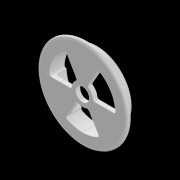
# Autodesk Inventor part: ToroidalCap
Saved by Autodesk Inventor 2020.4 (Build 244396010, 396A)
## iProperties
Created: 2022-09-18
Part Number: ToroidalCap
Material: Generic
Document SubType Name: Modeling
Designer: Val
Density: 1 g/cm^3
Appearance: Default
Author: Val
Autodesk Inventor part; units mm, degrees
ref_plane "YZ Plane" through (0, 0, 0) normal (1, 0, 0) x (0, 1, 0)
ref_plane "XZ Plane" through (0, 0, 0) normal (0, 1, 0) x (-1, 0, 0)
ref_plane "XY Plane" through (0, 0, 0) normal (0, 0, 1) x (1, 0, 0)
sketch "Sketch1" plane through (0, 0, 0) normal (0, 0, 1) x (1, 0, 0)
  circle A0 centre (0, 54.61) radius 54.61 construction
  circle A1 centre (0, 54.61) radius 42.291
  circle A2 centre (0, 54.61) radius 6.35
  circle A3 centre (0, 54.61) radius 44.45 construction
  circle A4 centre (0, 54.61) radius 35.1
  circle A5 centre (0, 54.61) radius 38.1 construction
  point P0 (0, 0)
  dimension "d1" = 12.7
  dimension "d60" = 3
  dimension "d61" = 84.582
  constraints: 6 centre point, 3 coincident, 4 other
  measures "d1" diameter of A2
  measures "d60" radial gap between concentric circles of A4 A5
  measures "d61" diameter of A1
extrude "Extrusion1" add sketch "Sketch1" along normal blind 4 contours A1 | A4
extrude "Extrusion2" add sketch "Sketch1" against normal blind 10 contours A4
sketch "Sketch2" plane through (0, 54.61, -10) normal (0, 0, -1) x (-1, 0, 0)
  circle A0 centre (0, 0) radius 35.1 projected
  circle A1 centre (0, 0) radius 6.35 projected
  circle A2 centre (0, 0) radius 6.35 projected
  circle A3 centre (0, 0) radius 31.1
  point P0 (0, -54.61)
  dimension "d7" = 4
  constraints: 1 centre point, 1 coincident
  measures "d7" radial gap between concentric circles of A3 A0
extrude "Extrusion3" cut sketch "Sketch2" against normal up to surface (10 mm away) contours A3
fillet "Fillet1" radius 2 2 edges at (-42.291, 54.61, 0) (-35.1, 54.61, -10)
fillet "Fillet2" radius 2 1 edges at (-42.291, 54.61, 4)
fillet "Fillet3" radius 2 2 edges at (-35.1, 54.61, 0) (31.1, 54.61, 0)
sketch "Sketch7" plane through (0, 54.61, 4) normal (0, 0, 1) x (1, 0, 0)
  spline S0 degree 3 poles (20.3422, -0.5357) (17.6586, -0.5357) (14.9744, -0.5026) (12.2915, -0.5485) (10.7524, -0.5749) (9.8489, -0.0663) (9.6665, 1.6089) (9.386, 4.1836) (8.1051, 6.2786) (6.0785, 7.8513) (5.077, 8.6285) (4.9277, 9.309) (5.5725, 10.41) (8.4292, 15.2878) (11.2449, 20.1902) (14.0203, 25.1147) (14.8305, 26.5522) (15.684, 26.6353) (16.9844, 25.7314) (25.3065, 19.9468) (29.8641, 12.0169) (30.8134, 1.9373) (30.9844, 0.1209) (30.4434, -0.6138) (28.6102, -0.5683) (25.8558, -0.5) (23.0984, -0.5505) (20.3422, -0.5505) (20.3422, -0.5456) (20.3422, -0.5407) (20.3422, -0.5357) knots 0 0 0 0 1 1 1 2 2 2 3 3 3 4 4 4 5 5 5 6 6 6 7 7 7 8 8 8 9 9 9 10 10 10 10
  line L0 (20.3422, -0.5357) -> (17.6586, -0.5357) construction
  line L1 (17.6586, -0.5357) -> (14.9744, -0.5026) construction
  line L2 (14.9744, -0.5026) -> (12.2915, -0.5485) construction
  line L3 (12.2915, -0.5485) -> (10.7524, -0.5749) construction
  line L4 (10.7524, -0.5749) -> (9.8489, -0.0663) construction
  line L5 (9.8489, -0.0663) -> (9.6665, 1.6089) construction
  line L6 (9.6665, 1.6089) -> (9.386, 4.1836) construction
  line L7 (9.386, 4.1836) -> (8.1051, 6.2786) construction
  line L8 (8.1051, 6.2786) -> (6.0785, 7.8513) construction
  line L9 (6.0785, 7.8513) -> (5.077, 8.6285) construction
  line L10 (5.077, 8.6285) -> (4.9277, 9.309) construction
  line L11 (4.9277, 9.309) -> (5.5725, 10.41) construction
  line L12 (5.5725, 10.41) -> (8.4292, 15.2878) construction
  line L13 (8.4292, 15.2878) -> (11.2449, 20.1902) construction
  line L14 (11.2449, 20.1902) -> (14.0203, 25.1147) construction
  line L15 (14.0203, 25.1147) -> (14.8305, 26.5522) construction
  line L16 (14.8305, 26.5522) -> (15.684, 26.6353) construction
  line L17 (15.684, 26.6353) -> (16.9844, 25.7314) construction
  line L18 (16.9844, 25.7314) -> (25.3065, 19.9468) construction
  line L19 (25.3065, 19.9468) -> (29.8641, 12.0169) construction
  line L20 (29.8641, 12.0169) -> (30.8134, 1.9373) construction
  line L21 (30.8134, 1.9373) -> (30.9844, 0.1209) construction
  line L22 (30.9844, 0.1209) -> (30.4434, -0.6138) construction
  line L23 (30.4434, -0.6138) -> (28.6102, -0.5683) construction
  line L24 (28.6102, -0.5683) -> (25.8558, -0.5) construction
  line L25 (25.8558, -0.5) -> (23.0984, -0.5505) construction
  line L26 (23.0984, -0.5505) -> (20.3422, -0.5505) construction
  line L27 (20.3422, -0.5505) -> (20.3422, -0.5456) construction
  line L28 (20.3422, -0.5456) -> (20.3422, -0.5407) construction
  line L29 (20.3422, -0.5407) -> (20.3422, -0.5357) construction
  spline S1 degree 3 poles (-20.5602, -0.5451) (-23.3112, -0.5437) (-26.0628, -0.5085) (-28.813, -0.5572) (-30.4043, -0.5853) (-31.0158, 0.0939) (-30.9106, 1.6746) (-30.2175, 12.0913) (-25.3046, 20.0286) (-16.8038, 25.8947) (-15.7132, 26.6474) (-14.9385, 26.4126) (-14.3143, 25.3297) (-11.3868, 20.2517) (-8.4306, 15.1896) (-5.5864, 10.0653) (-5.3297, 9.6027) (-5.5616, 8.4739) (-5.9721, 8.1022) (-8.133, 6.1458) (-9.8222, 3.9633) (-10.1251, 0.9673) (-10.2691, -0.4575) (-11.2491, -0.5389) (-12.3071, -0.543) (-15.0581, -0.5536) (-17.8092, -0.5466) (-20.5602, -0.5451) knots 0 0 0 0 1 1 1 2 2 2 3 3 3 4 4 4 5 5 5 6 6 6 7 7 7 8 8 8 9 9 9 9
  line L30 (-20.5602, -0.5451) -> (-23.3112, -0.5437) construction
  line L31 (-23.3112, -0.5437) -> (-26.0628, -0.5085) construction
  line L32 (-26.0628, -0.5085) -> (-28.813, -0.5572) construction
  line L33 (-28.813, -0.5572) -> (-30.4043, -0.5853) construction
  line L34 (-30.4043, -0.5853) -> (-31.0158, 0.0939) construction
  line L35 (-31.0158, 0.0939) -> (-30.9106, 1.6746) construction
  line L36 (-30.9106, 1.6746) -> (-30.2175, 12.0913) construction
  line L37 (-30.2175, 12.0913) -> (-25.3046, 20.0286) construction
  line L38 (-25.3046, 20.0286) -> (-16.8038, 25.8947) construction
  line L39 (-16.8038, 25.8947) -> (-15.7132, 26.6474) construction
  line L40 (-15.7132, 26.6474) -> (-14.9385, 26.4126) construction
  line L41 (-14.9385, 26.4126) -> (-14.3143, 25.3297) construction
  line L42 (-14.3143, 25.3297) -> (-11.3868, 20.2517) construction
  line L43 (-11.3868, 20.2517) -> (-8.4306, 15.1896) construction
  line L44 (-8.4306, 15.1896) -> (-5.5864, 10.0653) construction
  line L45 (-5.5864, 10.0653) -> (-5.3297, 9.6027) construction
  line L46 (-5.3297, 9.6027) -> (-5.5616, 8.4739) construction
  line L47 (-5.5616, 8.4739) -> (-5.9721, 8.1022) construction
  line L48 (-5.9721, 8.1022) -> (-8.133, 6.1458) construction
  line L49 (-8.133, 6.1458) -> (-9.8222, 3.9633) construction
  line L50 (-9.8222, 3.9633) -> (-10.1251, 0.9673) construction
  line L51 (-10.1251, 0.9673) -> (-10.2691, -0.4575) construction
  line L52 (-10.2691, -0.4575) -> (-11.2491, -0.5389) construction
  line L53 (-11.2491, -0.5389) -> (-12.3071, -0.543) construction
  line L54 (-12.3071, -0.543) -> (-15.0581, -0.5536) construction
  line L55 (-15.0581, -0.5536) -> (-17.8092, -0.5466) construction
  line L56 (-17.8092, -0.5466) -> (-20.5602, -0.5451) construction
  spline S2 degree 3 poles (-0.0271, -31.0202) (-4.7803, -30.8518) (-9.3441, -29.8755) (-13.6877, -27.8951) (-15.2539, -27.181) (-15.6734, -26.3929) (-14.6794, -24.7311) (-11.8581, -20.0145) (-9.2006, -15.1993) (-6.5165, -10.4017) (-5.9017, -9.3027) (-5.2264, -8.7506) (-3.9154, -9.3133) (-1.3197, -10.4273) (1.2719, -10.1999) (3.9287, -9.3573) (4.5356, -9.1649) (5.7982, -9.6542) (6.1334, -10.2082) (9.0163, -14.9731) (11.7012, -19.8576) (14.568, -24.6326) (15.5321, -26.2385) (15.1757, -27.0835) (13.6108, -27.8445) (9.2993, -29.9411) (4.7108, -30.7878) (-0.0271, -31.0202) knots 0 0 0 0 1 1 1 2 2 2 3 3 3 4 4 4 5 5 5 6 6 6 7 7 7 8 8 8 9 9 9 9
  line L57 (-0.0271, -31.0202) -> (-4.7803, -30.8518) construction
  line L58 (-4.7803, -30.8518) -> (-9.3441, -29.8755) construction
  line L59 (-9.3441, -29.8755) -> (-13.6877, -27.8951) construction
  line L60 (-13.6877, -27.8951) -> (-15.2539, -27.181) construction
  line L61 (-15.2539, -27.181) -> (-15.6734, -26.3929) construction
  line L62 (-15.6734, -26.3929) -> (-14.6794, -24.7311) construction
  line L63 (-14.6794, -24.7311) -> (-11.8581, -20.0145) construction
  line L64 (-11.8581, -20.0145) -> (-9.2006, -15.1993) construction
  line L65 (-9.2006, -15.1993) -> (-6.5165, -10.4017) construction
  line L66 (-6.5165, -10.4017) -> (-5.9017, -9.3027) construction
  line L67 (-5.9017, -9.3027) -> (-5.2264, -8.7506) construction
  line L68 (-5.2264, -8.7506) -> (-3.9154, -9.3133) construction
  line L69 (-3.9154, -9.3133) -> (-1.3197, -10.4273) construction
  line L70 (-1.3197, -10.4273) -> (1.2719, -10.1999) construction
  line L71 (1.2719, -10.1999) -> (3.9287, -9.3573) construction
  line L72 (3.9287, -9.3573) -> (4.5356, -9.1649) construction
  line L73 (4.5356, -9.1649) -> (5.7982, -9.6542) construction
  line L74 (5.7982, -9.6542) -> (6.1334, -10.2082) construction
  line L75 (6.1334, -10.2082) -> (9.0163, -14.9731) construction
  line L76 (9.0163, -14.9731) -> (11.7012, -19.8576) construction
  line L77 (11.7012, -19.8576) -> (14.568, -24.6326) construction
  line L78 (14.568, -24.6326) -> (15.5321, -26.2385) construction
  line L79 (15.5321, -26.2385) -> (15.1757, -27.0835) construction
  line L80 (15.1757, -27.0835) -> (13.6108, -27.8445) construction
  line L81 (13.6108, -27.8445) -> (9.2993, -29.9411) construction
  line L82 (9.2993, -29.9411) -> (4.7108, -30.7878) construction
  line L83 (4.7108, -30.7878) -> (-0.0271, -31.0202) construction
  spline S3 degree 3 poles (-0.0758, -5.9) (-3.1878, -5.905) (-5.9599, -3.1717) (-5.9422, -0.1159) (-5.9237, 3.0593) (-3.1623, 5.7847) (0.0741, 5.822) (3.0605, 5.8563) (5.8448, 2.9521) (5.7949, -0.1452) (5.7426, -3.392) (3.1893, -5.8948) (-0.0758, -5.9) knots 0 0 0 0 1 1 1 2 2 2 3 3 3 4 4 4 4
  line L84 (-0.0758, -5.9) -> (-3.1878, -5.905) construction
  line L85 (-3.1878, -5.905) -> (-5.9599, -3.1717) construction
  line L86 (-5.9599, -3.1717) -> (-5.9422, -0.1159) construction
  line L87 (-5.9422, -0.1159) -> (-5.9237, 3.0593) construction
  line L88 (-5.9237, 3.0593) -> (-3.1623, 5.7847) construction
  line L89 (-3.1623, 5.7847) -> (0.0741, 5.822) construction
  line L90 (0.0741, 5.822) -> (3.0605, 5.8563) construction
  line L91 (3.0605, 5.8563) -> (5.8448, 2.9521) construction
  line L92 (5.8448, 2.9521) -> (5.7949, -0.1452) construction
  line L93 (5.7949, -0.1452) -> (5.7426, -3.392) construction
  line L94 (5.7426, -3.392) -> (3.1893, -5.8948) construction
  line L95 (3.1893, -5.8948) -> (-0.0758, -5.9) construction
  circle A0 centre (0, 0) radius 6.35 projected
  point P0 (0, -54.61)
  constraints: 8 other
extrude "Extrusion8" cut sketch "Sketch7" against normal through all contours S0 | S1 | S2
body "Solid1"
